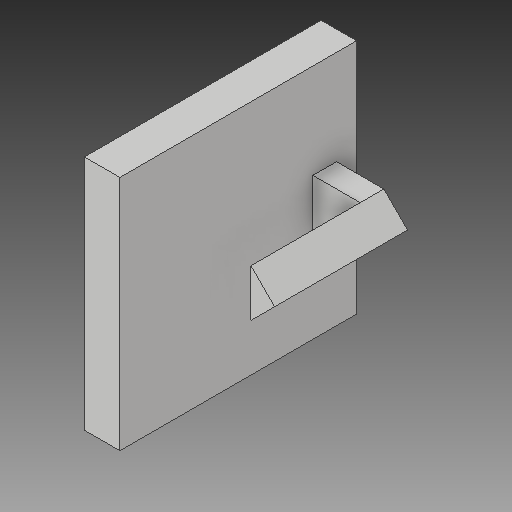
# Autodesk Inventor part: crochet
Saved by Autodesk Inventor 2017 (Build 210142000, 142)
## iProperties
Created: 2017-01-05
Part Number: crochet
Material: Generic
Document SubType Name: Modeling
Designer: Aegir
Density: 1 g/cm^3
Appearance: Default
Author: Aegir
Autodesk Inventor part; units mm, degrees
ref_plane "YZ Plane" through (0, 0, 0) normal (1, 0, 0) x (0, 1, 0)
ref_plane "XZ Plane" through (0, 0, 0) normal (0, 1, 0) x (-1, 0, 0)
ref_plane "XY Plane" through (0, 0, 0) normal (0, 0, 1) x (1, 0, 0)
sketch "Esquisse1" plane through (0, 0, 0) normal (1, 0, 0) x (0, 1, 0)
  line L0 (5.4849, 2.6087) -> (-4.5151, 2.6087)
  line L1 (-4.5151, 2.6087) -> (-4.5151, -7.3913)
  line L2 (-4.5151, -7.3913) -> (5.4849, -7.3913)
  line L3 (5.4849, -7.3913) -> (5.4849, 2.6087)
  point P0 (0, 0)
  dimension "d0" = 10
  dimension "d1" = 10
  constraints: 8 end point, 2 parallel, 1 horizontal, 1 perpendicular
  measures "d0" distance of L1.end L2.end
  measures "d1" distance of L2.end L0.start
extrude "Extrusion1" add sketch "Esquisse1" along normal blind 1.5
sketch "Esquisse2" plane through (1.5, 0, 0) normal (1, 0, 0) x (0, 0, -1)
  line L0 (5.5438, 1.4849) -> (6.5438, 1.4849)
  line L1 (6.5438, 1.4849) -> (6.5438, -0.5151)
  line L2 (6.5438, -0.5151) -> (5.5438, -0.5151)
  line L3 (5.5438, -0.5151) -> (5.5438, 1.4849)
  line L4 (7.3913, 5.4849) -> (-2.6087, 5.4849) projected
  point P0 (0, 0)
  dimension "d4" = 1
  dimension "d5" = 2
  dimension "d6" = 4
  constraints: 8 end point, 2 parallel, 1 horizontal, 1 perpendicular
  measures "d4" distance of L0.start L0.end
  measures "d5" distance of L2.end L0.start
  measures "d6" distance between parallel lines of L4 L0
extrude "Extrusion2" add sketch "Esquisse2" along normal blind 2
sketch "Esquisse3" plane through (3.5, 0, 0) normal (1, 0, 0) x (0, 0, -1)
  line L0 (6.5438, 1.4849) -> (6.5438, -0.5151) projected
  line L1 (6.5438, 1.4849) -> (0.9284, 1.4849)
  line L2 (0.9284, 1.4849) -> (0.9284, -0.5151)
  line L3 (0.9284, -0.5151) -> (6.5438, -0.5151)
  line L4 (6.5438, -0.5151) -> (6.5438, 1.4849)
  point P0 (0, 0)
  constraints: 8 end point, 2 parallel, 1 horizontal, 1 perpendicular
extrude "Extrusion3" add sketch "Esquisse3" along normal blind 1
chamfer "Chanfrein1" distance 1 angle 45 2 edges at (4.5, 1.4849, -3.7361) (4.5, -0.5151, -3.7361)
